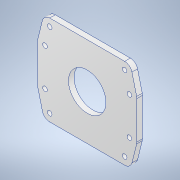
# Autodesk Inventor part: 関節3_775側_プーリ側板
Saved by Autodesk Inventor 2021 (Build 250183000, 183)
## iProperties
Created: 2022-01-31
Part Number: 関節3_775側_プーリ側板
Material: アルミニウム 6061
Document SubType Name: Modeling
Designer: hirohumi
Density: 2.7 g/cm^3
Appearance: アルミニウム - フラット
Author: hirohumi
Autodesk Inventor part; units mm, degrees
ref_plane "YZ Plane" through (0, 0, 0) normal (1, 0, 0) x (0, 1, 0)
ref_plane "XZ Plane" through (0, 0, 0) normal (0, 1, 0) x (-1, 0, 0)
ref_plane "XY Plane" through (0, 0, 0) normal (0, 0, 1) x (1, 0, 0)
sketch "スケッチ1" plane through (0, 0, 0) normal (0, 0, 1) x (1, 0, 0)
  circle A0 centre (0, 0) radius 10
  line L0 (22.5, 10) -> (-22.5, 10) construction
  line L1 (-22.5, 10) -> (-22.5, -10) construction
  line L2 (-22.5, -10) -> (22.5, -10) construction
  line L3 (22.5, -10) -> (22.5, 10) construction
  line L4 (22.5, 10) -> (-22.5, -10) construction
  line L5 (-22.5, 10) -> (22.5, -10) construction
  circle A1 centre (-22.5, 10) radius 1.25
  circle A2 centre (-22.5, -10) radius 1.25
  circle A3 centre (22.5, 10) radius 1.25
  circle A4 centre (22.5, -10) radius 1.25
  circle A5 centre (0, 0) radius 25 construction
  line L6 (20, 20) -> (-20, 20) construction
  line L7 (-20, 20) -> (-20, -20) construction
  line L8 (-20, -20) -> (20, -20) construction
  line L9 (20, -20) -> (20, 20) construction
  line L10 (20, 20) -> (-20, -20) construction
  line L11 (-20, 20) -> (20, -20) construction
  circle A6 centre (-20, 20) radius 1.25
  circle A7 centre (20, 20) radius 1.25
  circle A8 centre (20, -20) radius 1.25
  circle A9 centre (-20, -20) radius 1.25
  arc A10 (-20, 24) -> (-23.8806, 20.9701) centre (-20, 20) ccw
  arc A11 (-26.3806, 10.9701) -> (-26.5, 10) centre (-22.5, 10) ccw
  arc A12 (-26.5, -10) -> (-26.3806, -10.9701) centre (-22.5, -10) ccw
  arc A13 (-23.8806, -20.9701) -> (-20, -24) centre (-20, -20) ccw
  arc A14 (20, -24) -> (23.8806, -20.9701) centre (20, -20) ccw
  arc A15 (26.3806, -10.9701) -> (26.5, -10) centre (22.5, -10) ccw
  arc A16 (26.5, 10) -> (26.3806, 10.9701) centre (22.5, 10) ccw
  arc A17 (23.8806, 20.9701) -> (20, 24) centre (20, 20) ccw
  line L12 (-23.8806, 20.9701) -> (-26.3806, 10.9701)
  line L13 (-20, 24) -> (20, 24)
  line L14 (23.8806, 20.9701) -> (26.3806, 10.9701)
  line L15 (26.5, 10) -> (26.5, -10)
  line L16 (26.3806, -10.9701) -> (23.8806, -20.9701)
  line L17 (20, -24) -> (-20, -24)
  line L18 (-23.8806, -20.9701) -> (-26.3806, -10.9701)
  line L19 (-26.5, 10) -> (-26.5, -10)
  dimension "d0" = 20
  dimension "d1" = 45
  dimension "d2" = 20
  dimension "d3" = 2.5
  dimension "d4" = 2.5
  dimension "d5" = 2.5
  dimension "d6" = 2.5
  dimension "d7" = 50
  dimension "d8" = 40
  dimension "d9" = 40
  dimension "d10" = 2.5
  dimension "d11" = 2.5
  dimension "d12" = 2.5
  dimension "d13" = 2.5
  dimension "d14" = 4
  dimension "d15" = 4
  dimension "d16" = 4
  dimension "d17" = 4
  dimension "d18" = 4
  dimension "d19" = 4
  dimension "d20" = 4
  dimension "d21" = 4
  constraints: 40 end point, 18 centre point, 18 coincident, 16 point on circle, 14 tangent, 4 midpoint, 4 parallel, 3 horizontal, 3 perpendicular
  measures "d0" diameter of A0
  measures "d1" distance of L2.end L1.end
  measures "d2" distance of L1.end L0.end
  measures "d3" diameter of A1
  measures "d4" diameter of A2
  measures "d5" diameter of A3
  measures "d6" diameter of A4
  measures "d7" diameter of A5
  measures "d8" distance of L8.end L7.end
  measures "d9" distance of L7.end L6.end
  measures "d10" diameter of A6
  measures "d11" diameter of A7
  measures "d12" diameter of A8
  measures "d13" diameter of A9
  measures "d14" radius of A10
  measures "d15" radius of A17
  measures "d16" radius of A16
  measures "d17" radius of A15
  measures "d18" radius of A14
  measures "d19" radius of A13
  measures "d20" radius of A12
  measures "d21" radius of A11
extrude "押し出し1" add sketch "スケッチ1" along normal blind 3
